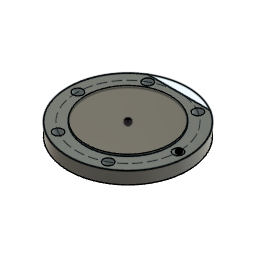
Cryo counterheater plate v1 (Autodesk Fusion 360 design; units mm, degrees)
Autodesk Fusion 360 part; units mm, degrees
sketch "Sketch1" plane through (0, 0, 0) normal (0, 1, 0) x (1, 0, 0)
  circle A0 centre (0, 0) radius 34
  line L0 (-17.7482, 29) -> (17.7482, 29)
  circle A1 centre (0, 0) radius 29 construction
  circle A2 centre (0, 0) radius 24
  point P0 (29, 0)
  dimension "d1" = 68
  dimension "d2" = 29
  dimension "d3" = 58
  dimension "d4" = 48
  constraint coincident A0.centre A1.centre
  constraint coincident A0 L0.start
  constraint coincident A0 L0.end
  constraint horizontal L0
  constraint concentric A0 A1
  constraint concentric A1 A2
  constraint coincident A1 P0
  constraint horizontal A0.centre P0
  measures "d1" diameter of A0
  measures "d2" distance of A0.centre L0
  measures "d3" diameter of A1
  measures "d4" diameter of A2
extrude "Extrude1" add sketch "Sketch1" against normal blind 7 contours A0 L0 | A2 picked at (0.5978, 27.311)
extrude "Extrude2" add sketch "Sketch1" along normal blind 1 contours A2
hole "Hole1" at (29, 0, 0.5) direction (0, -1, 0) diameter 5.5 end through all
pattern_circular "C-Pattern1" count 6 over 360 about axis through (0, 1.75, 0) along (0, 1, 0) of "Hole1"
sketch "Sketch2" plane through (0, 0, -29) normal (0, 0, -1) x (-1, 0, 0)
  line L0 (17.7482, 0) -> (-17.7482, 0)
  line L1 (-17.7482, 0) -> (-17.7482, -7)
  line L2 (-17.7482, -7) -> (17.7482, -7)
  line L3 (17.7482, -7) -> (17.7482, 0)
  line L4 (9, -3.5) -> (-7, -3.5) construction
  point P0 (9, -3.5)
  point P1 (-7, -3.5)
  dimension "d14" = 3.5
  constraint coincident P0 L4.start
  constraint coincident P1 L4.end
  constraint parallel L0 L4
  measures "d14" distance of L2 L4
hole "Hole2" at (-9, -3.5, -29) at (7, -3.5, -29) direction (0, 0, 1) diameter 1.623 depth 5 tip angle 118
thread "Thread1" "ISO Metric profile 2.0 M2x0.4 6H" thread offset 0 thread depth 10
equation "d4 = ( 24 * 2 ) * 1 mm"
